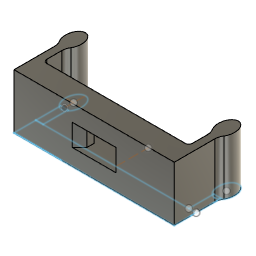
ender5-rail-clip (Autodesk Fusion 360 design; units mm, degrees)
Autodesk Fusion 360 part; units mm, degrees
note: some values were not read from the file. Set by a fixed rule: which sketch regions a step uses.
sketch "Sketch1" plane through (0, 0, 0) normal (0, 0, 1) x (1, 0, 0) in component "Ender5RailClip"
  line L0 (-21.0864, 9.1534) -> (22.9136, 9.1534)
  line L1 (22.9136, 9.1534) -> (22.9136, 3.1534)
  line L2 (22.9136, 3.1534) -> (-21.0864, 3.1534)
  line L3 (-21.0864, 3.1534) -> (-21.0864, 9.1534)
  line L4 (-21.0864, 9.1534) -> (-19.0864, 9.1534)
  line L5 (-19.0864, 9.1534) -> (-19.0864, 16)
  line L6 (-19.0864, 16) -> (-21.0864, 16)
  line L7 (-21.0864, 16) -> (-21.0864, 9.1534)
  line L8 (0.9136, 9.1534) -> (0.9136, 18) construction
  ellipse E0 centre (-20.0864, 18.5) end of major axis (-20.0864, 15.25) minor radius 2.2
  line L9 (-20.0864, 21.75) -> (-20.0864, 15.25)
  line L10 (-22.2864, 18.5) -> (-17.8864, 18.5)
  ellipse E1 centre (21.9136, 18.5) end of major axis (21.9136, 15.25) minor radius 2.2
  line L11 (20.9136, 16) -> (22.9136, 16)
  line L12 (20.9136, 9.1534) -> (20.9136, 16)
  line L13 (22.9136, 16) -> (22.9136, 9.1534)
  point P0 (-20.0864, 16)
  dimension "d2" = 6
  dimension "d3" = 2
  dimension "d4" = 6.5
  dimension "d5" = 4.4
  dimension "d6" = 2.5
  dimension "d19" = 40
  constraint horizontal L0
  constraint vertical L1
  constraint horizontal L2
  constraint vertical L3
  constraint horizontal L4
  constraint vertical L5
  constraint horizontal L6
  constraint vertical L7
  constraint midpoint L0 L8.start
  constraint perpendicular L0 L8
  constraint vertical L9
  constraint coincident E0 L9.start
  constraint coincident E0 L9.end
  constraint coincident E0 L10.start
  constraint coincident E0 L10.end
  constraint symmetric L0.start L8 L0.end
  constraint symmetric L4.end L8 L12.start
  constraint symmetric L5.end L8 L11.start
  constraint symmetric L6.end L8 L11.end
  constraint symmetric L8 E0 E1
  constraint midpoint L6 P0
  constraint vertical L9.end P0
  measures "d2" distance of L0.start L2.end
  measures "d3" distance of L0.start L4.end
  measures "d4" distance of E0
  measures "d6" distance of L6 E0.centre
  measures "d19" distance of L5 L12
extrude "Extrude1" add sketch "Sketch1" along normal blind 15 in component "Ender5RailClip"
fillet "Fillet1" radius 1 2 edges at (20.9136, 9.1534, 7.5) (-19.0864, 9.1534, 7.5) in component "Ender5RailClip"
fillet "Fillet2" radius 3.5 4 edges at (-19.0864, 15.6051, 7.5) (20.9136, 15.6051, 7.5) (-21.0864, 15.6051, 7.5) (22.9136, 15.6051, 7.5) in component "Ender5RailClip"
sketch "Sketch2" plane through (0, 3.1534, 0) normal (0, -1, 0) x (1, 0, 0) in component "Ender5RailClip"
  line L0 (-21.0864, 0) -> (22.9136, 0)
  line L1 (22.9136, 0) -> (22.9136, 15)
  line L2 (22.9136, 15) -> (-21.0864, 15)
  line L3 (-21.0864, 15) -> (-21.0864, 0)
  line L4 (0.9136, 0) -> (0.9136, 15) construction
  line L5 (-21.0864, 7.5) -> (22.9136, 7.5) construction
  line L6 (4.9136, 4.5) -> (-3.0864, 4.5)
  line L7 (-3.0864, 4.5) -> (-3.0864, 10.5)
  line L8 (-3.0864, 10.5) -> (4.9136, 10.5)
  line L9 (4.9136, 10.5) -> (4.9136, 4.5)
  line L10 (4.9136, 4.5) -> (-3.0864, 10.5) construction
  line L11 (-3.0864, 4.5) -> (4.9136, 10.5) construction
  point P0 (0.9136, 7.5)
  dimension "d20" = 8
  dimension "d21" = 6
  constraint midpoint L0 L4.start
  constraint midpoint L2 L4.end
  constraint midpoint L3 L5.start
  constraint midpoint L1 L5.end
  constraint horizontal L6
  constraint perpendicular L6 L7
  constraint parallel L6 L8
  constraint parallel L7 L9
  constraint coincident L10 P0
  constraint coincident L11 P0
  constraint midpoint L4 P0
  measures "d20" distance of L7.end L8.end
  measures "d21" distance of L6.end L7.end
extrude "Extrude3" cut sketch "Sketch2" against normal through all contours L6 L7 L8 L9 in component "Ender5RailClip"
chamfer "Chamfer2" distance 2 angle 45 4 edges at (-3.0864, 9.1534, 7.5) (-3.0864, 3.1534, 7.5) (4.9136, 9.1534, 7.5) (4.9136, 3.1534, 7.5) in component "Ender5RailClip"
component "Ender5RailClip" placed x (1, 0, 0) y (0, 1, 0) z (0, 0, 1) at (0, 0, 0)
